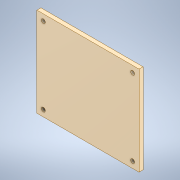
# Autodesk Inventor part: 8020_Base_Tx_Filter_v1
Saved by Autodesk Inventor 2021 (Build 250183000, 183)
## iProperties
Created: 2021-03-01
Part Number: 8020_Base_Tx_Filter_v1
Material: Polyethylene, High Density
Document SubType Name: Modeling
Designer: Barksdale
Density: 0.952 g/cm^3
Appearance: Smooth - Off-White
Author: Barksdale
Autodesk Inventor part; units mm, degrees
ref_plane "YZ Plane" through (0, 0, 0) normal (1, 0, 0) x (0, 1, 0)
ref_plane "XZ Plane" through (0, 0, 0) normal (0, 1, 0) x (-1, 0, 0)
ref_plane "XY Plane" through (0, 0, 0) normal (0, 0, 1) x (1, 0, 0)
sketch "Sketch1" plane through (0, 0, 0) normal (0, 0, 1) x (1, 0, 0)
  line L0 (0, 0) -> (160, 0)
  line L1 (160, 0) -> (160, 140)
  line L2 (160, 140) -> (0, 140)
  line L3 (0, 140) -> (0, 0)
  dimension "d0" = 160
  dimension "d1" = 140
  constraints: 8 end point, 2 parallel, 1 horizontal, 1 perpendicular
  measures "d0" distance of L2.end L1.end
  measures "d1" distance of L0.end L1.end
extrude "Extrusion1" add sketch "Sketch1" along normal blind 6.3
sketch "Sketch2" plane through (0, 0, 6.3) normal (0, 0, 1) x (1, 0, 0)
  line L0 (0, 0) -> (10, 0)
  line L1 (10, 0) -> (10, 10)
  line L2 (10, 10) -> (0, 10)
  line L3 (0, 10) -> (0, 0)
  line L4 (0, 140) -> (0, 0) projected
  line L5 (0, 140) -> (10, 140)
  line L6 (10, 140) -> (10, 130)
  line L7 (10, 130) -> (0, 130)
  line L8 (0, 130) -> (0, 140)
  line L9 (160, 0) -> (160, 140) projected
  line L10 (160, 140) -> (150, 140)
  line L11 (150, 140) -> (150, 130)
  line L12 (150, 130) -> (160, 130)
  line L13 (160, 130) -> (160, 140)
  line L14 (160, 0) -> (150, 0)
  line L15 (150, 0) -> (150, 10)
  line L16 (150, 10) -> (160, 10)
  line L17 (160, 10) -> (160, 0)
  line L18 (10, 10) -> (10, 10)
  line L19 (10, 10) -> (10, 10)
  line L20 (10, 10) -> (10, 10)
  line L21 (10, 10) -> (10, 10)
  circle A0 centre (10, 130) radius 3.175
  circle A1 centre (150, 130) radius 3.175
  circle A2 centre (150, 10) radius 3.175
  circle A3 centre (10, 10) radius 3.175
  dimension "d4" = 10
  dimension "d5" = 10
  dimension "d6" = 10
  dimension "d7" = 10
  dimension "d8" = 10
  dimension "d9" = 10
  dimension "d10" = 10
  dimension "d11" = 10
  dimension "d12" = 0
  dimension "d13" = 0
  dimension "d14" = 6.35
  dimension "d15" = 6.35
  dimension "d16" = 6.35
  dimension "d17" = 6.35
  constraints: 40 end point, 10 equal length, 5 horizontal, 5 perpendicular, 4 centre point, 4 coincident
  measures "d4" distance of L2.end L1.end
  measures "d5" distance of L1.end L0.end
  measures "d6" distance of L6.end L7.end
  measures "d7" distance of L5.end L6.end
  measures "d8" distance of L12.end L11.end
  measures "d9" distance of L11.end L10.end
  measures "d10" distance of L15.end L16.end
  measures "d11" distance of L14.end L15.end
  measures "d12" distance of L20.end L19.end
  measures "d13" distance of L19.end L18.end
  measures "d14" diameter of A0
  measures "d15" diameter of A1
  measures "d16" diameter of A2
  measures "d17" diameter of A3
extrude "Extrusion2" cut sketch "Sketch2" against normal blind 10 contours A3 L2 L1 | L1 L2 A3 | A0 L6 L7 | L7 L6 A0 | A2 L15 L16 | L16 L15 A2 | A1 L11 L12 | L12 L11 A1
body "Solid1"
